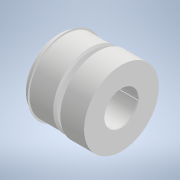
# Autodesk Inventor part: 71. Блок шестерен заднего хода
Saved by Autodesk Inventor 2021 (Build 250183000, 183)
## iProperties
Created: 2021-03-23
Part Number: 71. Блок шестерен заднего хода
Material: Типовые
Document SubType Name: Modeling
Designer: Данил
Density: 1 g/cm^3
Appearance: По умолчанию
Author: Данил
Autodesk Inventor part; units mm, degrees
ref_plane "YZ Plane" through (0, 0, 0) normal (1, 0, 0) x (0, 1, 0)
ref_plane "XZ Plane" through (0, 0, 0) normal (0, 1, 0) x (-1, 0, 0)
ref_plane "XY Plane" through (0, 0, 0) normal (0, 0, 1) x (1, 0, 0)
sketch "Эскиз1" plane through (0, 0, 0) normal (0, 0, 1) x (1, 0, 0)
  line L0 (-26.5, 0) -> (26.5, 0)
  line L1 (-26.5, -14.3929) -> (-26.5, -27.5)
  line L2 (-25.5, -28.5) -> (-24, -28.5)
  line L3 (-26.5, -14.3929) -> (-25.5, -14.125)
  line L4 (-25.5, -14.125) -> (25.5, -14.125)
  line L5 (-25.5, -28.5) -> (-26.5, -27.5)
  line L6 (-21, -31.5) -> (-21, -36.75)
  arc A0 (-21, -31.5) -> (-24, -28.5) centre (-24, -31.5) ccw
  line L7 (-21, -36.75) -> (-0.5, -36.75)
  line L8 (-0.5, -36.75) -> (-0.5, -30.5)
  line L9 (-0.5, -30.5) -> (1, -29)
  line L10 (1, -29) -> (1, -23)
  line L11 (1, -23) -> (5, -23)
  line L12 (5, -23) -> (5, -29)
  line L13 (5, -29) -> (6.5, -30.5)
  line L14 (6.5, -30.5) -> (6.5, -45.125)
  line L15 (6.5, -45.125) -> (26.5, -45.125)
  line L16 (26.5, -45.125) -> (26.5, -14.3929)
  line L17 (26.5, -14.3929) -> (25.5, -14.125)
  point P0 (0, 0)
  point P1 (0, 0)
  point P2 (-26.5, -28.5)
  dimension "d0" = 53
  dimension "d1" = 28.25
  dimension "d2" = 15
  dimension "d3" = 57
  dimension "d4" = 1
  dimension "d5" = 1
  dimension "d6" = 45
  dimension "d7" = 3
  dimension "d8" = 73.5
  dimension "d9" = 5.5
  dimension "d10" = 7
  dimension "d11" = 4
  dimension "d12" = 46
  dimension "d13" = 21.5
  dimension "d14" = 20
  dimension "d15" = 58
  dimension "d16" = 45
  dimension "d17" = 15
  dimension "d18" = 1
  dimension "d19" = 90.25
  constraints: 36 end point, 5 perpendicular, 4 horizontal, 3 vertical, 2 parallel, 2 point on circle, 2 point on line, 2 tangent, 2 vertical alignment, 1 centre point, 1 coincident, 1 horizontal alignment, 1 midpoint
  measures "d0" distance of L0.start L0.end
  measures "d1" diameter of L4 L0
  measures "d2" angle of L4 L3
  measures "d3" diameter of L2 L0
  measures "d4" distance from line of L1 L3.end
  measures "d5" distance of L2.start point (-26.5, -28.5)
  measures "d6" angle of L2 L5
  measures "d7" radius of A0
  measures "d8" diameter of L7 L0
  measures "d9" distance from line of L0.start L6
  measures "d10" distance between parallel lines of L8 L14
  measures "d11" distance of L10.end L11.end
  measures "d12" diameter of L11 L0
  measures "d13" distance from line of L0.end L12
  measures "d14" distance from line of L0.end L14
  measures "d15" diameter of L9.end L0
  measures "d16" angle of L8 L9
  measures "d17" angle of L4 L17
  measures "d18" horizontal distance of L4.end L16.end
  measures "d19" diameter of L15 L0
revolve "Вращение1" add sketch "Эскиз1" angle 360 about axis through (-26.5, 0, 0) along (1, 0, 0)
sketch "Эскиз2" plane through (0, 0, 0) normal (0, 0, 1) x (1, 0, 0)
  line L0 (26.5, 45.125) -> (6.5, 45.125) projected
  line L1 (26.5, 0) -> (6.5, 0)
  line L2 (26.5, 45.125) -> (26.5, -45.125) projected
  line L3 (6.5, 45.125) -> (26.5, 45.125)
  line L4 (26.5, 45.125) -> (26.5, 31.5)
  line L5 (26.5, 31.5) -> (6.5, 31.5)
  line L6 (6.5, 31.5) -> (6.5, 45.125)
  point P0 (0, 0)
  dimension "d21" = 63
  constraints: 10 end point, 2 horizontal, 2 parallel, 2 vertical alignment, 1 horizontal alignment, 1 perpendicular, 1 point on line
  measures "d21" diameter of L5 L1
revolve "Вращение2" cut sketch "Эскиз2" angle 360 about axis through (26.5, 0, 0) along (-1, 0, 0)
fillet "Сопряжение1" radius 0.75 2 edges at (1, 23, 0) (5, 23, 0)
sketch "Эскиз3" plane through (0, 0, 0) normal (0, 0, 1) x (1, 0, 0)
  line L0 (-21, 36.75) -> (-21, -36.75) projected
  line L1 (-0.5, 36.75) -> (-0.5, -36.75) projected
  line L2 (-21, 31.5) -> (-21, -31.5) projected
  line L3 (-21, 0) -> (0, 0)
  line L4 (-21, 36.75) -> (-0.5, 36.75)
  line L5 (-0.5, 36.75) -> (-0.5, 30)
  line L6 (-0.5, 30) -> (-21, 30)
  line L7 (-21, 30) -> (-21, 36.75)
  point P0 (-21, 30)
  dimension "d24" = 60
  constraints: 10 end point, 2 parallel, 2 perpendicular, 1 horizontal, 1 midpoint, 1 point on line
  measures "d24" diameter of L6 L3
revolve "Вращение3" cut sketch "Эскиз3" angle 360 about axis through (-21, 0, 0) along (1, 0, 0) contours L4 L1 L6 L0
sketch "Эскиз4" plane through (-26.5, 0, 0) normal (-1, 0, 0) x (0, 0, 1)
  line L0 (-14.5451, 1.5) -> (-14.0451, 1.5)
  line L1 (-14.0451, 1.5) -> (-14.0451, -1.5)
  line L2 (-14.0451, -1.5) -> (-14.5451, -1.5)
  line L3 (-14.5451, -1.5) -> (-14.5451, 1.5)
  circle A0 centre (0, 0) radius 14.125 projected
  point P0 (0, 0)
  point P1 (-14.0451, 0)
  dimension "d26" = 3
  dimension "d27" = 0.5
  constraints: 8 end point, 2 parallel, 1 horizontal, 1 horizontal alignment, 1 midpoint, 1 perpendicular, 2 other
  measures "d26" distance of L0.end L1.end
  measures "d27" distance of L1.end L2.end
extrude "Выдавливание1" cut sketch "Эскиз4" against normal through all contours L0 A0 L2 L3 | L1 A0 picked at (-14.0688, 0.1669)
mirror "Зеркальное отражение1" about plane through (0, 0, 0) normal (0, 0, 1) of "Выдавливание1"
